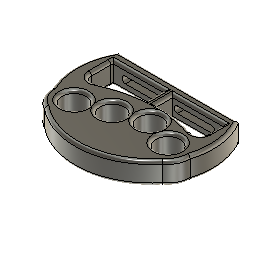
Knuckles v4 (Autodesk Fusion 360 design; units mm, degrees)
Autodesk Fusion 360 part; units mm, degrees
sketch "Sketch1" plane through (0, 0, 0) normal (0, 0, 1) x (1, 0, 0)
  line L0 (-80, 0) -> (-77.3049, 0)
  line L1 (-77.3049, 0) -> (106.9178, 0) construction
  line L2 (0, 0) -> (0, 50) construction
  circle A0 centre (0, 50) radius 12
  line L3 (-11.9987, 50.176) -> (-27.9987, 50.176) construction
  line L4 (-27.9987, 50.176) -> (-27.9987, 40.176) construction
  circle A1 centre (-27.9987, 40.176) radius 12
  line L5 (-27.9987, 40.176) -> (-55.9987, 40.176) construction
  line L6 (-55.9987, 40.176) -> (-55.9987, 30.176) construction
  circle A2 centre (-55.9987, 30.176) radius 12
  line L7 (0, 50) -> (28, 50) construction
  line L8 (28, 50) -> (28, 40)
  circle A3 centre (28, 40) radius 12
  circle A4 centre (-55.9987, 30.176) radius 22
  circle A5 centre (28, 40) radius 22
  arc A6 (50, 40.0331) -> (-77.9973, 30.4264) centre (-15.8418, 59.7872) ccw
  line L9 (53.7496, 94.1084) -> (-91.2504, 94.1084)
  arc A7 (-75.714, 20.4134) -> (49.7632, 36.7806) centre (-18.2002, 68.6521) ccw
  dimension "d1" = 50
  dimension "d2" = 24
  dimension "d3" = 16
  dimension "d4" = 10
  dimension "d5" = 24
  dimension "d6" = 28
  dimension "d7" = 10
  dimension "d8" = 24
  dimension "d9" = 28
  dimension "d10" = 10
  dimension "d11" = 24
  dimension "d12" = 10
  dimension "d13" = 10
  constraint horizontal L0
  constraint parallel L0 L1
  constraint coincident L2.start origin
  constraint perpendicular L1 L2
  constraint coincident L2.end A0.centre
  constraint coincident A0 L3.start
  constraint perpendicular L2 L3
  constraint perpendicular L3 L4
  constraint coincident L4.end A1.centre
  constraint perpendicular L4 L5
  constraint perpendicular L5 L6
  constraint coincident L6.end A2.centre
  constraint perpendicular L2 L7
  constraint perpendicular L7 L8
  constraint coincident L8.end A3.centre
  constraint coincident A5 A6.start
  constraint coincident A4 A6.end
  constraint horizontal L9
  constraint coincident A5 A7.end
  constraint coincident A4 A7.start
  measures "d1" distance of L2.start L2.end
  measures "d2" diameter of A0
  measures "d3" distance of L3.start L3.end
  measures "d4" distance of L3.end L4.end
  measures "d5" diameter of A1
  measures "d6" distance of L4.end L5.end
  measures "d7" distance of L5.end L6.end
  measures "d8" diameter of A2
  measures "d9" distance of L2.end L7.end
  measures "d10" distance of L7.end L8.end
  measures "d11" diameter of A3
extrude "Extrude1" add sketch "Sketch1" along normal blind 22 contours A0 A5 A7 | A0 A1 A4 A5 A6 L9 A7 | A5 A7 | A1 A4 A7 | A4 A7
sketch "Sketch2" plane through (0, 0, 22) normal (0, 0, 1) x (-1, 0, 0)
  circle A0 centre (55.9987, -30.176) radius 12
  arc A1 (70.7651, -83.8525) -> (83.9886, -30.7457) centre (16.0375, -42.0258) ccw
  arc A2 (83.9886, -30.7457) -> (67.2324, -14.1943) centre (67.9987, -30.176) ccw
  arc A3 (67.2324, -14.1943) -> (-32.101, -24.1131) centre (25.257, -96.1797) ccw
  arc A4 (-32.101, -24.1131) -> (-49.9999, -39.932) centre (-34, -40) ccw
  arc A5 (-49.9999, -39.932) -> (-39.2782, -84.4747) centre (17.727, -47.1916) ccw
  line L0 (-39.2782, -84.4747) -> (70.7651, -83.8525)
  arc A6 (-50.2229, -51.9284) -> (84.8878, -39.9694) centre (8.5285, 53.5165) ccw
  line L1 (15.7434, -84.1636) -> (15.6068, -60.0057) construction
  line L2 (19.7434, -84.141) -> (19.6068, -59.9831)
  line L3 (11.7435, -84.1862) -> (11.6069, -60.0284)
  line L4 (70.8894, -45) -> (70.8894, -84.2528)
  line L5 (-39.3602, -55) -> (-39.3602, -85.2147)
  circle A7 centre (0, -50) radius 12
  circle A8 centre (27.9987, -40.176) radius 12
  circle A9 centre (-28, -40) radius 12
  arc A10 (77.9973, -30.4264) -> (65.4095, -10.2904) centre (55.9987, -30.176) ccw
  arc A11 (65.4095, -10.2904) -> (-40.5565, -21.9353) centre (18.2002, -68.6521) ccw
  arc A12 (-40.5565, -21.9353) -> (-50, -40.0331) centre (-28, -40) ccw
  arc A13 (-50, -40.0331) -> (-43.7184, -94.1084) centre (15.8418, -59.7872) ccw
  line L6 (-43.7184, -94.1084) -> (75.4019, -94.1084)
  arc A14 (75.4019, -94.1084) -> (77.9973, -30.4264) centre (15.8418, -59.7872) ccw
  dimension "d38" = 4
  dimension "d39" = -4
  constraint coincident A5 A6.start
  constraint coincident A1 A6.end
  constraint midpoint L0 L1.start
  constraint perpendicular L0 L1
  constraint vertical L4
  constraint vertical L5
extrude "Extrude5" cut sketch "Sketch2" against normal blind 50 contours A1 L0 A6 L2 L4 | A5 L0 A6 L3 L5
sketch "Sketch5" plane through (0, 94.1084, 0) normal (0, 1, 0) x (-1, 0, 0)
  line L0 (-43.7184, 0) -> (75.4019, 0)
  line L1 (75.4019, 0) -> (75.4019, 22)
  line L2 (75.4019, 22) -> (-43.7184, 22)
  line L3 (-43.7184, 22) -> (-43.7184, 0)
  line L4 (-43.7184, 11) -> (75.4019, 11) construction
  line L5 (15.8418, 22) -> (15.8418, 0) construction
  line L6 (11.7435, 0) -> (11.7435, 22)
  line L7 (11.6472, 22) -> (11.6472, 0)
  line L8 (19.6446, 0) -> (19.6446, 22)
  line L9 (19.7434, 22) -> (19.7434, 0)
  line L10 (-26.899, 7.7244) -> (7.0112, 7.7244)
  arc A0 (7.0112, 7.7244) -> (7.0112, 14.2756) centre (7.0112, 11) ccw
  line L11 (7.0112, 14.2756) -> (-26.899, 14.2756)
  arc A1 (-26.899, 14.2756) -> (-26.899, 7.7244) centre (-26.899, 11) ccw
  line L12 (-30.1745, 11) -> (10.2868, 11) construction
  line L13 (58.5825, 7.7244) -> (24.6723, 7.7244)
  arc A2 (24.6723, 14.2756) -> (24.6723, 7.7244) centre (24.6723, 11) ccw
  line L14 (24.6723, 14.2756) -> (58.5825, 14.2756)
  arc A3 (58.5825, 7.7244) -> (58.5825, 14.2756) centre (58.5825, 11) ccw
  line L15 (11.6472, 0) -> (11.7435, 0)
  line L16 (11.7435, 22) -> (11.6472, 22)
  line L17 (19.7434, 0) -> (19.6446, 0)
  line L18 (19.6446, 22) -> (19.7434, 22)
  point P0 (-39.2782, 22)
  point P1 (70.7651, 22)
  constraint midpoint L3 L4.start
  constraint midpoint L1 L4.end
  constraint midpoint L2 L5.start
  constraint midpoint L0 L5.end
  constraint tangent L10 A0
  constraint tangent A0 L11
  constraint parallel L10 L11
  constraint tangent L11 A1
  constraint tangent L10 A1
  constraint midpoint A1 L12.start
  constraint midpoint A0 L12.end
  constraint coincident L4 L12.end
  constraint perpendicular L6 L12
  constraint symmetric L5 L10.start L13.start
  constraint symmetric L5 L10.end L13.end
  constraint symmetric L5 A0.end A2.start
  constraint symmetric L5 L11.end L14.end
  constraint symmetric L5 A0 A2
  constraint symmetric L5 A1 A3
extrude "Extrude6" cut sketch "Sketch5" against normal blind 15 contours L10 A0 L11 A1 | L13 A2 L14 A3
fillet "Fillet6" radius 7.5 1 edges at (39.3602, 57.2852, 11)
fillet "Fillet7" radius 7.5 1 edges at (-70.8894, 49.8347, 11)
fillet "Fillet8" radius 12.5 1 edges at (39.3602, 84.3491, 11)
fillet "Fillet9" radius 20 1 edges at (-70.8894, 83.6894, 11)
sketch "Sketch6" plane through (0, 0, 22) normal (0, 0, 1) x (-1, 0, 0)
  circle A0 centre (55.9987, -30.176) radius 12
  arc A1 (-39.3602, -83.0457) -> (-39.2782, -84.4747) centre (-26.8602, -83.0457) ccw
  arc A2 (-29.4975, -61.0452) -> (11.6472, -67.1509) centre (8.5285, 53.5165) ccw
  line L0 (11.6472, -67.1509) -> (11.7435, -84.1862)
  line L1 (11.7435, -84.1862) -> (-39.2782, -84.4747)
  line L2 (70.7651, -83.8525) -> (19.7434, -84.141)
  line L3 (19.7434, -84.141) -> (19.6446, -66.6783)
  arc A3 (19.6446, -66.6783) -> (60.1801, -55.5819) centre (8.5285, 53.5165) ccw
  arc A4 (70.8894, -62.3606) -> (60.1801, -55.5819) centre (63.3894, -62.3606) ccw
  line L4 (70.8894, -62.3606) -> (70.8894, -81.6262)
  arc A5 (70.7651, -83.8525) -> (70.8894, -81.6262) centre (50.8894, -81.6262) ccw
  circle A6 centre (0, -50) radius 12
  circle A7 centre (27.9987, -40.176) radius 12
  circle A8 centre (-28, -40) radius 12
  arc A9 (77.9973, -30.4264) -> (65.4095, -10.2904) centre (55.9987, -30.176) ccw
  arc A10 (65.4095, -10.2904) -> (-40.5565, -21.9353) centre (18.2002, -68.6521) ccw
  arc A11 (-40.5565, -21.9353) -> (-50, -40.0331) centre (-28, -40) ccw
  arc A12 (-50, -40.0331) -> (-43.7184, -94.1084) centre (15.8418, -59.7872) ccw
  line L5 (-43.7184, -94.1084) -> (75.4019, -94.1084)
  arc A13 (75.4019, -94.1084) -> (77.9973, -30.4264) centre (15.8418, -59.7872) ccw
  line L6 (-39.3602, -83.0457) -> (-39.3602, -68.1633)
  arc A14 (-29.4975, -61.0452) -> (-39.3602, -68.1633) centre (-31.8602, -68.1633) ccw
extrude "Extrude7" [suppressed]
fillet "Fillet10" radius 3 1 faces at (-4.7814, 22.5197, 22)
fillet "Fillet11" radius 3 1 faces at (-4.7814, 22.5197, 0)
equation "d3 = 12 mm + 4 mm"
equation "d6 = 24 mm + 4 mm"
equation "d9 = 24 mm + 4 mm"
